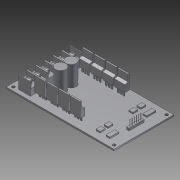
# Autodesk Inventor part: MotorDriver
Saved by Autodesk Inventor 2011 SP2 (Build 150309200, 309)
## iProperties
Created: 2015-09-17
Part Number: MotorDriver
Document SubType Name: Modeling
Designer: Ernest
Density: 1 g/cm^3
Author: Ernest
Autodesk Inventor part; units mm, degrees
ref_plane "YZ Plane" through (0, 0, 0) normal (1, 0, 0) x (0, 1, 0)
ref_plane "XZ Plane" through (0, 0, 0) normal (0, 1, 0) x (-1, 0, 0)
ref_plane "XY Plane" through (0, 0, 0) normal (0, 0, 1) x (1, 0, 0)
sketch "Sketch1" plane through (0, 0, 0) normal (0, 0, 1) x (1, 0, 0)
  line L0 (-54.075, -30) -> (54.075, -30)
  line L1 (54.075, -30) -> (54.075, 30)
  line L2 (54.075, 30) -> (-54.075, 30)
  line L3 (-54.075, 30) -> (-54.075, -30)
  point P0 (0, 0)
  dimension "d0" = 108.15
  dimension "d1" = 54.075
  dimension "d2" = 60
  dimension "d3" = 30
  constraints: 8 end point, 2 parallel, 1 horizontal, 1 perpendicular
  measures "d0" distance of L0.start L0.end
  measures "d1" distance from line of point (0, 0) L3
  measures "d2" distance of L0.end L1.end
  measures "d3" distance from line of point (0, 0) L0
extrude "Extrusion1" add sketch "Sketch1" along normal blind 1.6
sketch "Sketch2" plane through (0, 0, 1.6) normal (0, 0, 1) x (1, 0, 0)
  line L0 (-54.075, -30) -> (-54.075, 30) projected
  line L1 (54.075, -30) -> (-54.075, -30) projected
  line L2 (54.075, 30) -> (54.075, -30) projected
  line L3 (-54.075, 30) -> (54.075, 30) projected
  circle A0 centre (-50.575, 26.35) radius 1.5
  circle A1 centre (-50.575, -26.35) radius 1.5
  circle A2 centre (50.575, 26.35) radius 1.5
  circle A3 centre (50.575, -26.35) radius 1.5
  line L4 (43.375, 8.6) -> (45.875, 8.6)
  line L5 (45.875, 8.6) -> (45.875, -6.7)
  line L6 (45.875, -6.7) -> (43.375, -6.7)
  line L7 (43.375, -6.7) -> (43.375, 8.6)
  line L8 (39.075, 23) -> (43.075, 23)
  line L9 (43.075, 23) -> (43.075, 14)
  line L10 (43.075, 14) -> (39.075, 14)
  line L11 (39.075, 14) -> (39.075, 23)
  line L12 (39.075, -14) -> (43.075, -14)
  line L13 (43.075, -14) -> (43.075, -23)
  line L14 (43.075, -23) -> (39.075, -23)
  line L15 (39.075, -23) -> (39.075, -14)
  line L16 (29.075, 23) -> (33.075, 23)
  line L17 (33.075, 23) -> (33.075, 18)
  line L18 (33.075, 18) -> (29.075, 18)
  line L19 (29.075, 18) -> (29.075, 23)
  line L20 (29.075, 15) -> (33.075, 15)
  line L21 (33.075, 15) -> (33.075, 10)
  line L22 (33.075, 10) -> (29.075, 10)
  line L23 (29.075, 10) -> (29.075, 15)
  line L24 (29.075, -18) -> (33.075, -18)
  line L25 (33.075, -18) -> (33.075, -23)
  line L26 (33.075, -23) -> (29.075, -23)
  line L27 (29.075, -23) -> (29.075, -18)
  line L28 (29.075, -10) -> (33.075, -10)
  line L29 (33.075, -10) -> (33.075, -15)
  line L30 (33.075, -15) -> (29.075, -15)
  line L31 (29.075, -15) -> (29.075, -10)
  line L32 (-45.625, 26) -> (-33.725, 26)
  line L33 (-33.725, 26) -> (-33.725, -26)
  line L34 (-33.725, -26) -> (-45.625, -26)
  line L35 (-45.625, -26) -> (-45.625, 26)
  line L36 (-31.125, -21.125) -> (14.875, -21.125)
  line L37 (14.875, -21.125) -> (14.875, -21.725)
  line L38 (14.875, -21.725) -> (-31.125, -21.725)
  line L39 (-31.125, -21.725) -> (-31.125, -21.125)
  line L40 (-31.125, 21.725) -> (14.875, 21.725)
  line L41 (14.875, 21.725) -> (14.875, 21.125)
  line L42 (14.875, 21.125) -> (-31.125, 21.125)
  line L43 (-31.125, 21.125) -> (-31.125, 21.725)
  line L44 (-45.625, 25.35) -> (-33.725, 25.35)
  line L45 (-45.625, -25.35) -> (-33.725, -25.35)
  line L46 (-45.625, 0.63) -> (-33.725, 0.63)
  line L47 (-33.725, -0.67) -> (-45.625, -0.67)
  line L48 (-45.625, 8.03) -> (-33.725, 8.03)
  line L49 (-33.725, 9.33) -> (-45.625, 9.33)
  line L50 (-45.625, 16.69) -> (-33.725, 16.69)
  line L51 (-33.725, 17.99) -> (-45.625, 17.99)
  line L52 (-45.625, -8.03) -> (-33.725, -8.03)
  line L53 (-33.725, -9.33) -> (-45.625, -9.33)
  line L54 (-45.625, -16.69) -> (-33.725, -16.69)
  line L55 (-33.725, -17.99) -> (-45.625, -17.99)
  circle A4 centre (-24.275, -5.225) radius 5.15
  circle A5 centre (-24.275, 5.225) radius 5.15
  point P0 (0, 0)
  dimension "d6" = 3
  dimension "d7" = 3
  dimension "d8" = 3
  dimension "d9" = 3
  dimension "d10" = 2.15
  dimension "d11" = 2
  dimension "d12" = 2
  dimension "d13" = 2
  dimension "d15" = 2
  dimension "d16" = 2.15
  dimension "d17" = 2.15
  dimension "d18" = 2.15
  dimension "d19" = 52
  dimension "d20" = 11.9
  dimension "d21" = 8.45
  dimension "d22" = 4
  dimension "d23" = 0.6
  dimension "d24" = 0.6
  dimension "d25" = 2.6
  dimension "d27" = 43.45
  dimension "d28" = 8.275
  dimension "d29" = 4
  dimension "d30" = 5
  dimension "d31" = 21.4
  dimension "d32" = 15.3
  dimension "d33" = 2.5
  dimension "d34" = 25
  dimension "d35" = 15
  dimension "d36" = 7
  dimension "d37" = 7
  dimension "d38" = 46
  dimension "d39" = 4
  dimension "d40" = 9
  dimension "d41" = 7
  dimension "d42" = 7
  dimension "d43" = 3
  dimension "d44" = 3
  dimension "d45" = 8.2
  dimension "d48" = 1.3
  dimension "d49" = 1.3
  dimension "d50" = 1.3
  dimension "d51" = 0.65
  dimension "d52" = 1.3
  dimension "d53" = 1.3
  dimension "d54" = 0.65
  dimension "d55" = 7.36
  dimension "d56" = 7.36
  dimension "d57" = 7.36
  dimension "d58" = 7.36
  dimension "d59" = 7.36
  dimension "d148" = 4.3
  dimension "d149" = 4.3
  dimension "d150" = 10.3
  dimension "d151" = 10.3
  dimension "d152" = 10.45
  dimension "d153" = 24.775
  constraints: 100 end point, 23 horizontal, 19 parallel, 9 perpendicular, 8 equal length, 6 centre point, 6 collinear, 30 other
  measures "d6" diameter of A0
  measures "d7" diameter of A1
  measures "d8" diameter of A2
  measures "d9" diameter of A3
  measures "d10" distance edge to line of A1 L1
  measures "d11" distance edge to line of A1 L0
  measures "d12" distance edge to line of A0 L0
  measures "d13" distance edge to line of A2 L2
  measures "d15" distance edge to line of A3 L2
  measures "d16" distance edge to line of A3 L1
  measures "d17" distance edge to line of A2 L3
  measures "d18" distance edge to line of A0 L3
  measures "d19" distance of L34.end L32.start
  measures "d20" distance of L34.start L34.end
  measures "d22" distance between parallel lines of L32 L3
  measures "d23" distance of L36.end L37.end
  measures "d24" distance of L40.end L41.end
  measures "d27" distance between parallel lines of L38 L40
  measures "d28" distance between parallel lines of L1 L38
  measures "d29" distance of L16.start L16.end
  measures "d30" distance of L18.end L16.start
  measures "d31" distance between parallel lines of L4 L3
  measures "d32" distance of L4.end L5.end
  measures "d33" distance of L5.end L6.end
  measures "d34" distance between parallel lines of L2 L19
  measures "d35" distance between parallel lines of L2 L11
  measures "d36" distance between parallel lines of L3 L8
  measures "d37" distance between parallel lines of L1 L14
  measures "d38" distance of L40.start L40.end
  measures "d39" distance of L9.end L10.end
  measures "d40" distance of L8.end L9.end
  measures "d41" distance between parallel lines of L3 L16
  measures "d42" distance between parallel lines of L1 L26
  measures "d43" distance between parallel lines of L30 L24
  measures "d44" distance between parallel lines of L20 L18
  measures "d45" distance between parallel lines of L2 L5
  measures "d48" distance between parallel lines of L47 L46
  measures "d49" distance between parallel lines of L48 L49
  measures "d50" distance between parallel lines of L50 L51
  measures "d51" distance between parallel lines of L44 L32
  measures "d52" distance between parallel lines of L53 L52
  measures "d53" distance between parallel lines of L55 L54
  measures "d54" distance between parallel lines of L34 L45
  measures "d55" distance between parallel lines of L55 L45
  measures "d56" distance between parallel lines of L51 L44
  measures "d57" distance between parallel lines of L49 L50
  measures "d58" distance between parallel lines of L53 L54
  measures "d59" distance between parallel lines of L47 L52
  measures "d150" diameter of A4
  measures "d151" diameter of A5
  measures "d152" distance of A5.centre A4.centre
  measures "d153" distance from line of A4.centre L1
extrude "Extrusion2" cut sketch "Sketch2" against normal up to next contours A0 | A1 | A2 | A3
extrude "Extrusion3" add sketch "Sketch2" along normal blind 12.5 contours L32 L33 L44 L35 | L51 L33 L50 L35 | L49 L33 L48 L35 | L46 L33 L47 L35 | L52 L33 L53 L35 | L54 L33 L55 L35 | L45 L33 L34 L35
extrude "Extrusion4" add sketch "Sketch2" along normal blind 6.6 contours L44 L33 L51 L35 | L50 L33 L49 L35 | L48 L33 L46 L35 | L47 L33 L52 L35 | L53 L33 L54 L35 | L55 L33 L45 L35
sketch "Sketch3" plane through (0, 0, 8.2) normal (0, 0, 1) x (1, 0, 0)
  line L0 (-33.725, -9.33) -> (-33.725, -16.69) projected
  line L1 (-45.625, -9.33) -> (-33.725, -9.33) projected
  line L2 (-45.625, -16.69) -> (-45.625, -9.33) projected
  line L3 (-33.725, -16.69) -> (-45.625, -16.69) projected
  line L4 (-45.625, -25.35) -> (-45.625, -17.99) projected
  line L5 (-33.725, -25.35) -> (-45.625, -25.35) projected
  line L6 (-33.725, -17.99) -> (-33.725, -25.35) projected
  line L7 (-45.625, -17.99) -> (-33.725, -17.99) projected
  line L8 (-45.625, 0.63) -> (-45.625, 8.03) projected
  line L9 (-33.725, 0.63) -> (-45.625, 0.63) projected
  line L10 (-33.725, 8.03) -> (-33.725, 0.63) projected
  line L11 (-45.625, 8.03) -> (-33.725, 8.03) projected
  line L12 (-33.725, 9.33) -> (-45.625, 9.33) projected
  line L13 (-33.725, 16.69) -> (-33.725, 9.33) projected
  line L14 (-45.625, 16.69) -> (-33.725, 16.69) projected
  line L15 (-45.625, 9.33) -> (-45.625, 16.69) projected
  line L16 (-45.625, 25.35) -> (-33.725, 25.35) projected
  line L17 (-45.625, 17.99) -> (-45.625, 25.35) projected
  line L18 (-33.725, 17.99) -> (-45.625, 17.99) projected
  line L19 (-33.725, 25.35) -> (-33.725, 17.99) projected
  circle A0 centre (-39.675, -21.67) radius 2.5
  circle A1 centre (-39.675, -13.01) radius 2.5
  circle A2 centre (-39.675, -4.35) radius 2.5
  circle A3 centre (-39.675, 4.33) radius 2.5
  circle A4 centre (-39.675, 13.01) radius 2.5
  circle A5 centre (-39.675, 21.67) radius 2.5
  point P0 (0, 0)
  dimension "d64" = 5
  dimension "d65" = 5
  dimension "d66" = 5
  dimension "d67" = 5
  dimension "d68" = 5
  dimension "d69" = 5
  constraints: 6 centre point
  measures "d64" diameter of A0
  measures "d65" diameter of A1
  measures "d66" diameter of A2
  measures "d67" diameter of A3
  measures "d68" diameter of A4
  measures "d69" diameter of A5
extrude "Extrusion5" add sketch "Sketch3" along normal blind 4 contours A0 | A1 | A2 | A3 | A4 | A5
fillet "Fillet1" radius 2 6 edges at (-42.175, -21.67, 12.2) (-42.175, -13.01, 12.2) (-42.175, -4.35, 12.2) (-42.175, 4.33, 12.2) (-42.175, 13.01, 12.2) (-42.175, 21.67, 12.2)
extrude "Extrusion6" add sketch "Sketch2" along normal blind 4.35 contours L36 L37 L38 L39 | L40 L41 L42 L43
sketch "Sketch4" plane through (0, 0, 5.95) normal (0, 0, 1) x (1, 0, 0)
  line L0 (14.875, -21.125) -> (14.875, -21.725) projected
  line L1 (-31.125, -21.125) -> (14.875, -21.125) projected
  line L2 (-31.125, -21.725) -> (-31.125, -21.125) projected
  line L3 (14.875, 21.725) -> (14.875, 21.125) projected
  line L4 (-31.125, 21.725) -> (14.875, 21.725) projected
  line L5 (-31.125, 21.125) -> (-31.125, 21.725) projected
  line L6 (14.875, 21.125) -> (-31.125, 21.125) projected
  line L7 (14.875, -20.125) -> (-31.125, -20.125)
  line L8 (-31.125, -20.125) -> (-31.125, -24.575)
  line L9 (-31.125, -24.575) -> (14.875, -24.575)
  line L10 (14.875, -24.575) -> (14.875, -20.125)
  line L11 (-31.125, 20.125) -> (14.875, 20.125)
  line L12 (14.875, 20.125) -> (14.875, 24.575)
  line L13 (14.875, 24.575) -> (-31.125, 24.575)
  line L14 (-31.125, 24.575) -> (-31.125, 20.125)
  line L15 (14.875, 21.725) -> (14.875, 21.125) projected
  line L16 (-31.125, 21.125) -> (-31.125, 21.725) projected
  point P0 (0, 0)
  dimension "d75" = 4.45
  dimension "d76" = 1
  dimension "d77" = 1
  dimension "d78" = 4.45
  constraints: 16 end point, 4 collinear, 4 parallel, 2 horizontal, 2 perpendicular
  measures "d75" distance between parallel lines of L9 L7
  measures "d76" distance between parallel lines of L7 L1
  measures "d77" distance between parallel lines of L6 L11
  measures "d78" distance between parallel lines of L13 L11
extrude "Extrusion7" add sketch "Sketch4" along normal blind 14.55
sketch "Sketch5" plane through (14.875, -21.725, 1.6) normal (1, 0, 0) x (0, 0, -1)
  line L0 (-18.9, 1.6) -> (-18.9, -2.85) projected
  line L1 (-4.35, -2.85) -> (-18.9, -2.85) projected
  line L2 (0, 42.85) -> (-4.35, 42.85) projected
  line L3 (0, 43.45) -> (0, 42.85) projected
  line L4 (0, 43.45) -> (-4.35, 43.45) projected
  line L5 (-4.35, 43.45) -> (-4.35, 46.3) projected
  line L6 (-4.35, 46.3) -> (-18.9, 46.3) projected
  line L7 (-18.9, 46.3) -> (-18.9, 41.85) projected
  line L8 (-4.35, 41.85) -> (-18.9, 41.85) projected
  line L9 (-4.35, 41.85) -> (-4.35, 42.85) projected
  line L10 (-18.9, -1.55) -> (-12.25, -1.55)
  line L11 (-12.25, -1.55) -> (-11.406, 1.6)
  line L12 (-4.35, 1.6) -> (-18.9, 1.6) projected
  line L13 (-18.9, 46.3) -> (-18.9, 41.85) projected
  line L14 (-18.9, 45) -> (-12.25, 45)
  line L15 (-12.25, 45) -> (-11.406, 41.85)
  line L16 (-4.35, 41.85) -> (-18.9, 41.85) projected
  point P0 (1.6, 21.725)
  dimension "d81" = 6.65
  dimension "d82" = 105
  dimension "d83" = 1.3
  dimension "d84" = 105
  dimension "d85" = 1.3
  constraints: 8 end point, 4 point on line, 1 parallel, 1 perpendicular
  measures "d81" distance of L10.start L10.end
  measures "d82" angle of L11 L10
  measures "d83" distance between parallel lines of L1 L10
  measures "d84" angle of L14 L15
  measures "d85" distance between parallel lines of L14 L6
extrude "Extrusion8" cut sketch "Sketch5" against normal up to next contours L12 L11 L10 L0 | L8 L7 L14 L15
sketch "Sketch6" plane through (-31.125, -24.575, 5.95) normal (0, -1, 0) x (1, 0, 0)
  line L0 (46, 14.55) -> (0, 14.55) projected
  line L1 (0, 0) -> (0, 14.55) projected
  line L2 (0, 0) -> (46, 0) projected
  line L3 (46, 0) -> (46, 14.55) projected
  line L4 (46, 0) -> (0, 0) projected
  line L5 (0, -4.35) -> (0, 0) projected
  line L6 (46, -4.35) -> (0, -4.35) projected
  line L7 (46, -4.35) -> (46, 0) projected
  line L8 (10.3, 14.55) -> (10.3, -4.35)
  line L9 (46, -4.35) -> (0, -4.35) projected
  line L10 (11.9, 14.55) -> (11.9, -4.35)
  line L11 (22.2, 14.55) -> (22.2, -4.35)
  line L12 (35.7, 14.55) -> (35.7, -4.35)
  line L13 (34.1, 14.55) -> (34.1, -4.35)
  line L14 (23.8, 14.55) -> (23.8, -4.35)
  line L15 (46, 0) -> (0, 0) projected
  line L16 (44.5, 0) -> (44.5, -4.35)
  line L17 (42.95, 0) -> (42.95, -4.35)
  line L18 (41.625, 0) -> (41.625, -4.35)
  line L19 (40.075, 0) -> (40.075, -4.35)
  line L20 (38.75, 0) -> (38.75, -4.35)
  line L21 (37.2, 0) -> (37.2, -4.35)
  line L22 (32.6, 0) -> (32.6, -4.35)
  line L23 (31.05, 0) -> (31.05, -4.35)
  line L24 (29.725, 0) -> (29.725, -4.35)
  line L25 (28.175, 0) -> (28.175, -4.35)
  line L26 (26.85, 0) -> (26.85, -4.35)
  line L27 (25.3, 0) -> (25.3, -4.35)
  line L28 (13.4, 0) -> (13.4, -4.35)
  line L29 (14.95, 0) -> (14.95, -4.35)
  line L30 (16.275, 0) -> (16.275, -4.35)
  line L31 (17.825, 0) -> (17.825, -4.35)
  line L32 (19.15, 0) -> (19.15, -4.35)
  line L33 (20.7, 0) -> (20.7, -4.35)
  line L34 (8.8, 0) -> (8.8, -4.35)
  line L35 (7.25, 0) -> (7.25, -4.35)
  line L36 (5.925, 0) -> (5.925, -4.35)
  line L37 (4.375, 0) -> (4.375, -4.35)
  line L38 (1.5, 0) -> (1.5, -4.35)
  line L39 (3.05, 0) -> (3.05, -4.35)
  point P0 (31.125, -5.95)
  dimension "d88" = 10.3
  dimension "d89" = 1.6
  dimension "d90" = 1.6
  dimension "d91" = 1.6
  dimension "d92" = 10.3
  dimension "d93" = 10.3
  dimension "d99" = 1.5
  dimension "d101" = 1.5
  dimension "d106" = 1.55
  dimension "d107" = 1.55
  dimension "d108" = 1.55
  dimension "d109" = 1.325
  dimension "d110" = 1.5
  dimension "d111" = 1.5
  dimension "d112" = 1.55
  dimension "d113" = 1.55
  dimension "d114" = 1.325
  dimension "d115" = 1.55
  dimension "d116" = 1.55
  dimension "d117" = 1.55
  dimension "d118" = 1.55
  dimension "d119" = 1.55
  dimension "d120" = 1.55
  dimension "d121" = 1.55
  dimension "d122" = 1.5
  dimension "d123" = 1.5
  dimension "d124" = 1.325
  dimension "d125" = 1.5
  dimension "d126" = 1.5
  dimension "d127" = 1.325
  constraints: 60 end point, 22 perpendicular, 6 point on line, 5 parallel, 3 vertical, 56 other
  measures "d88" distance between parallel lines of L3 L12
  measures "d89" distance between parallel lines of L13 L12
  measures "d90" distance between parallel lines of L11 L14
  measures "d91" distance between parallel lines of L10 L8
  measures "d92" distance between parallel lines of L8 L1
  measures "d93" distance between parallel lines of L11 L10
  measures "d99" distance between parallel lines of L21 L12
  measures "d101" distance between parallel lines of L16 L7
  measures "d106" distance between parallel lines of L20 L21
  measures "d107" distance between parallel lines of L18 L19
  measures "d108" distance between parallel lines of L17 L16
  measures "d109" distance between parallel lines of L19 L20
  measures "d110" distance between parallel lines of L13 L22
  measures "d111" distance between parallel lines of L14 L27
  measures "d112" distance between parallel lines of L26 L27
  measures "d113" distance between parallel lines of L24 L25
  measures "d114" distance between parallel lines of L25 L26
  measures "d115" distance between parallel lines of L22 L23
  measures "d116" distance between parallel lines of L39 L38
  measures "d117" distance between parallel lines of L36 L37
  measures "d118" distance between parallel lines of L34 L35
  measures "d119" distance between parallel lines of L29 L28
  measures "d120" distance between parallel lines of L32 L33
  measures "d121" distance between parallel lines of L30 L31
  measures "d122" distance between parallel lines of L38 L5
  measures "d123" distance between parallel lines of L8 L34
  measures "d124" distance between parallel lines of L36 L35
  measures "d125" distance between parallel lines of L28 L10
  measures "d126" distance between parallel lines of L11 L33
  measures "d127" distance between parallel lines of L31 L32
extrude "Extrusion9" cut sketch "Sketch6" against normal through all contours L12 L2 L13 L0 | L7 L6 L16 L2 | L12 L6 L13 L2 | L2 L21 L6 L12 | L14 L2 L11 L0 | L13 L6 L22 L2 | L17 L6 L18 L2 | L14 L6 L11 L2 | L2 L27 L6 L14 | L2 L19 L6 L20 | L10 L2 L8 L0 | L11 L6 L33 L2 | L23 L6 L24 L2 | L10 L6 L8 L2 | L2 L28 L6 L10 | L2 L25 L6 L26 | L8 L6 L34 L2 | L32 L6 L31 L2 | L2 L38 L6 L5 | L2 L30 L6 L29 | L35 L6 L36 L2 | L2 L37 L6 L39
extrude "Extrusion10" add sketch "Sketch2" along normal blind 2.5 contours L4 L5 L6 L7
sketch "Sketch7" plane through (0, 0, 4.1) normal (0, 0, 1) x (1, 0, 0)
  line L0 (43.375, 8.6) -> (45.875, 8.6) projected
  circle A0 centre (44.625, 6.415) radius 0.3
  circle A1 centre (44.625, 4.229) radius 0.3
  circle A2 centre (44.625, 2.044) radius 0.3
  circle A3 centre (44.625, -0.142) radius 0.3
  circle A4 centre (44.625, -2.328) radius 0.3
  circle A5 centre (44.625, -4.514) radius 0.3
  point P0 (0, 0)
  dimension "d132" = 2.185
  dimension "d133" = 2.186
  dimension "d134" = 2.185
  dimension "d135" = 2.186
  dimension "d136" = 2.186
  dimension "d137" = 2.186
  dimension "d138" = 0.6
  dimension "d139" = 0.6
  dimension "d140" = 0.6
  dimension "d141" = 0.6
  dimension "d142" = 0.6
  dimension "d143" = 0.6
  constraints: 6 centre point
  measures "d132" distance from line of A0.centre L0
  measures "d133" distance of A1.centre A0.centre
  measures "d134" distance of A1.centre A2.centre
  measures "d135" distance of A3.centre A2.centre
  measures "d136" distance of A4.centre A3.centre
  measures "d137" distance of A5.centre A4.centre
  measures "d138" diameter of A0
  measures "d139" diameter of A1
  measures "d140" diameter of A2
  measures "d141" diameter of A3
  measures "d142" diameter of A4
  measures "d143" diameter of A5
extrude "Extrusion11" add sketch "Sketch7" along normal blind 5.9
extrude "Extrusion12" add sketch "Sketch2" along normal blind 1.5 contours L8 L9 L10 L11 | L12 L13 L14 L15 | L16 L17 L18 L19 | L20 L21 L22 L23 | L24 L25 L26 L27 | L28 L29 L30 L31
extrude "Extrusion13" add sketch "Sketch2" along normal blind 20.4 contours A4 | A5
body "Solid1"
